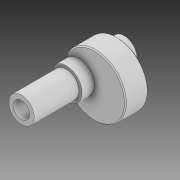
# Autodesk Inventor part: camshaft
Saved by Autodesk Inventor 2020 (Build 240168000, 168)
## iProperties
Created: 2020-11-25
Part Number: camshaft
Material: Generic
Document SubType Name: Modeling
Designer: DDeGo
Density: 1 g/cm^3
Appearance: Default
Author: DDeGo
Autodesk Inventor part; units mm, degrees
ref_plane "YZ Plane" through (0, 0, 0) normal (1, 0, 0) x (0, 1, 0)
ref_plane "XZ Plane" through (0, 0, 0) normal (0, 1, 0) x (-1, 0, 0)
ref_plane "XY Plane" through (0, 0, 0) normal (0, 0, 1) x (1, 0, 0)
sketch "Sketch1" plane through (0, 0, 0) normal (0, 0, 1) x (1, 0, 0)
  circle A0 centre (0, 0) radius 5.925
  dimension "d0" = 11.85
  constraints: 1 centre point, 1 coincident
  measures "d0" diameter of A0
extrude "Extrusion1" add sketch "Sketch1" along normal blind 4.4
chamfer "Chamfer1" distance 0.2 angle 45 2 edges at (-5.925, 0, 0) (-5.925, 0, 4.4)
sketch "Sketch2" plane through (0, 0, 4.4) normal (0, 0, 1) x (1, 0, 0)
  line L0 (0, 0) -> (-3, 0) construction
  circle A0 centre (-3, 0) radius 2.45
  dimension "d3" = 4.9
  dimension "d4" = 3
  constraints: 2 end point, 1 centre point, 1 coincident, 1 horizontal
  measures "d3" diameter of A0
  measures "d4" distance of L0.start L0.end
extrude "Extrusion2" add sketch "Sketch2" along normal blind 11
sketch "Sketch3" plane through (0, 0, 4.4) normal (0, 0, 1) x (1, 0, 0)
  circle A0 centre (-3, 0) radius 2.45 projected
  circle A1 centre (-3, 0) radius 3
  point P0 (0, 0)
  dimension "d7" = 6
  constraints: 1 centre point, 1 coincident
  measures "d7" diameter of A1
extrude "Extrusion3" add sketch "Sketch3" along normal blind 2.4 and the other way blind 1.1
sketch "Sketch4" plane through (0, 0, 0) normal (0, 0, -1) x (-1, 0, 0)
  circle A0 centre (3, 0) radius 2.45 projected
  point P0 (0, 0)
extrude "Extrusion4" add sketch "Sketch4" along normal blind 4.3 and the other way blind 1.5
sketch "Sketch5" plane through (0, 0, 0) normal (0, 0, -1) x (-1, 0, 0)
  circle A0 centre (3, 0) radius 3 projected
  point P0 (0, 0)
extrude "Extrusion5" add sketch "Sketch5" along normal blind 1.3 and the other way blind 1
sketch "Sketch7" plane through (-3, 0, 15.4) normal (0, 0, 1) x (1, 0, 0)
  circle A0 centre (0, 0) radius 2.45 construction
  circle A1 centre (0, 0) radius 1.575
  point P0 (3, 0)
  dimension "d25" = 3.15
  constraints: 1 centre point, 1 coincident
  measures "d25" diameter of A1
extrude "Extrusion7" cut sketch "Sketch7" against normal through all
sketch "Sketch8" plane through (-3, 0, 15.4) normal (0, 0, 1) x (1, 0, 0)
  line L0 (-2.3324, 4.9065) -> (-4.551, 4.9065)
  line L1 (-4.551, 4.9065) -> (-4.551, -6.3773)
  line L2 (-4.551, -6.3773) -> (-2.3324, -6.3773)
  line L3 (-2.3324, -6.3773) -> (-2.3324, 4.9065)
  circle A0 centre (0, 0) radius 2.45 construction
  line L4 (-2.45, -0.7065) -> (-2.45, 0.5926) construction
  circle A1 centre (0, 0) radius 2.45 projected
  point P0 (3, 0)
  point P1 (-2.3324, 0.75)
  point P2 (-2.3324, -0.75)
  dimension "d31" = 1.5
  constraints: 10 end point, 2 parallel, 2 point on circle, 2 point on line, 1 horizontal, 1 perpendicular, 1 tangent, 1 vertical
  measures "d31" distance of A1.end A1.start
extrude "Extrusion8" cut sketch "Sketch8" against normal through all contours L3 A1 L2 L1 L0 | L3 A1 picked at (-2.3672, 0.0845)
sketch "Sketch6" plane through (-3, 0, -4.3) normal (0, 0, -1) x (-1, 0, 0)
  circle A0 centre (0, 0) radius 2.5 projected
  point P0 (-3, 0)
body "Solid1"
